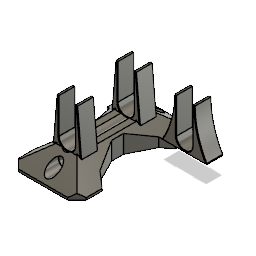
PlayStation TV Display Stand v8 (Autodesk Fusion 360 design; units mm, degrees)
Autodesk Fusion 360 part; units mm, degrees
(part 1 of 2)
sketch "Sketch1" plane through (0, 0, 0) normal (0, 0, 1) x (1, 0, 0)
  line L0 (0, 0) -> (14, 0)
  line L1 (14, 0) -> (14, 35)
  line L2 (14, 35) -> (0, 35)
  line L3 (0, 35) -> (0, 0)
  circle A0 centre (7, 7) radius 7
  line L4 (16, -2) -> (16, 37)
  line L5 (16, 37) -> (-2, 37)
  line L6 (-2, 37) -> (-2, -2)
  line L7 (-2, -2) -> (16, -2)
  line L8 (-2, 35) -> (16, 35)
  dimension "d1" = 14
  dimension "d2" = 35
  dimension "d3" = 2
  constraint horizontal L0
  constraint vertical L1
  constraint horizontal L2
  constraint vertical L3
  constraint coincident L0.start L3.end
  constraint tangent L0 A0
  constraint tangent L1 A0
  constraint tangent L3 A0
  constraint coincident L6 L8.start
  constraint coincident L4 L8.end
  constraint perpendicular L4 L8
  measures "d1" distance of L0.start L0.end
  measures "d2" distance of L0.start L2.end
extrude "Extrude1" add sketch "Sketch1" along normal blind 15 contours L0 L3 A0 | L0 L1 L3 L4 L6 L7 L8 | L0 L1 A0 makes body 1
extrude "Extrude2" add 1 faces at (4, -2, 5) along direction (0, -1, 0) blind 10 on bodies 1 bodies 1
extrude "Extrude3" add 1 faces at (4, -12, 5) along direction (0, -1, 0) blind 5 on bodies 1 bodies 1
sketch "Sketch2" plane through (0, 0, 15) normal (0, 0, 1) x (1, 0, 0)
  line L0 (16, -17) -> (16, 35)
  line L1 (16, 35) -> (14, 35)
  line L2 (14, 35) -> (14, 7)
  arc A0 (0, 7) -> (14, 7) centre (7, 7) ccw
  line L3 (0, 7) -> (0, 35)
  line L4 (0, 35) -> (-2, 35)
  line L5 (-2, 35) -> (-2, -17)
  line L6 (7, 0) -> (7, -4.4)
  circle A1 centre (7, -7) radius 2.6
  line L7 (7, -9.6) -> (7, -14)
  line L8 (16, -17) -> (-2, -17)
  line L9 (-2, -17) -> (-2, -14)
  line L10 (-2, -14) -> (16, -14)
  line L11 (16, -14) -> (16, -17)
  dimension "d10" = 4.4
  dimension "d27" = 5.2
  dimension "d28" = 4.4
  constraint midpoint A0 L6.start
  constraint vertical L6
  constraint coincident L6.end A1
  constraint coincident A1 L7.start
  constraint vertical L7
  constraint horizontal L8
  constraint vertical L9
  constraint horizontal L10
  constraint vertical L11
  constraint coincident L5 L9.end
  constraint coincident L0.start L8.start
  measures "d10" distance of L6.start L6.end
  measures "d27" diameter of A1
  measures "d28" distance of L7.start L7.end
extrude "Extrude4" cut sketch "Sketch2" against normal blind 36 contours L0 L5 L8 L9 L10 L11 bodies 1
sketch "Sketch3" plane through (0, -14, 0) normal (0, -1, 0) x (1, 0, 0)
  line L0 (-2, 0) -> (16, 0)
  line L1 (16, 0) -> (16, 15)
  line L2 (16, 15) -> (-2, 15)
  line L3 (-2, 15) -> (-2, 0)
  line L4 (-2, 7.5) -> (16, 7.5)
  line L5 (7, 7.5) -> (7, 9.3)
  line L6 (7, 9.3) -> (11.6, 9.3)
  line L7 (11.6, 9.3) -> (2.4, 9.3)
  line L8 (2.4, 9.3) -> (2.4, 5.7)
  line L9 (2.4, 5.7) -> (11.6, 5.7)
  line L10 (11.6, 5.7) -> (11.6, 9.3)
  line L11 (-2, 0) -> (16, 0)
  line L12 (16, 0) -> (16, 15)
  line L13 (16, 15) -> (-2, 15)
  line L14 (-2, 15) -> (-2, 0)
  dimension "d15" = 1.8
  dimension "d16" = 4.6
  dimension "d17" = 9.2
  dimension "d18" = 3.6
  constraint midpoint L3 L4.start
  constraint midpoint L1 L4.end
  constraint midpoint L4 L5.start
  constraint perpendicular L4 L5
  constraint perpendicular L5 L6
  constraint horizontal L7
  constraint vertical L8
  constraint horizontal L9
  constraint vertical L10
  measures "d15" distance of L5.start L5.end
  measures "d16" distance of L5.end L6.end
  measures "d17" distance of L6.end L7.end
  measures "d18" distance of L6.end L9.end
extrude "Extrude5" cut sketch "Sketch3" against normal blind 12 contours L4 L5 L7 L8 | L4 L8 L9 L10 | L4 L5 L6 L7 L10 bodies 1
extrude "Extrude9" cut sketch "Sketch2" against normal blind 25 contours A1 bodies 1
extrude "Extrude7" add 1 faces at (-0.6667, 35, 10) along direction (0, 1, 0) blind 2 on bodies 1 bodies 1
extrude "Extrude8" add 1 faces at (15.3333, 35, 10) along direction (0, 1, 0) blind 2 on bodies 1 bodies 1
sketch "Sketch14" plane through (0, 0, 5.7) normal (0, 0, 1) x (1, 0, 0)
  circle A0 centre (7, -7) radius 2.6
  line L0 (2.4, -14) -> (11.6, -14)
  line L1 (11.6, -14) -> (11.6, -2)
  line L2 (11.6, -2) -> (2.4, -2)
  line L3 (2.4, -2) -> (2.4, -14)
  line L4 (2.4, -14) -> (11.6, -14)
  line L5 (11.6, -14) -> (11.6, -2)
  line L6 (11.6, -2) -> (2.4, -2)
  line L7 (2.4, -2) -> (2.4, -14)
  circle A1 centre (7, -7) radius 2.6
  line L8 (3.2, -13.2) -> (10.8, -13.2)
  line L9 (10.8, -13.2) -> (10.8, -2.8)
  line L10 (10.8, -2.8) -> (3.2, -2.8)
  line L11 (3.2, -2.8) -> (3.2, -13.2)
  dimension "d133" = -0.8
  constraint horizontal L4
  constraint vertical L5
  constraint horizontal L6
  constraint vertical L7
  constraint coincident L1.end L2.start
  constraint coincident L0.start L3.end
  constraint concentric A0 A1
extrude "Extrude33" cut sketch "Sketch14" against normal blind 1.2 contours L8 L9 L10 L11 bodies 1
chamfer "Chamfer9" distance 1.2 distance2 3 1 edges at (7, -2.8, 4.5) measured on face at (8.2667, -2.8, 5.3) on bodies 1
chamfer "Chamfer10" distance 1.2 distance2 5 1 edges at (7, -13.2, 4.5) measured on face at (5.7333, -13.2, 5.3) on bodies 1
chamfer "Chamfer11" distance 1.2 distance2 1.49 2 edges at (10.8, -7, 4.5) (3.2, -7, 4.5) measured on face at (10.8, -8.0667, 5.3) measured on face at (3.2, -8.0667, 5.3) on bodies 1
copy_body "CopyPasteBodies1" bodies 1 makes body 2
move_body "Move1" bodies 2 to x (-1, 0, 0) y (0, 1, 0) z (0, 0, -1) at (14, 0, 95.1)
sketch "Sketch4" plane through (0, -14, 0) normal (0, -1, 0) x (1, 0, 0)
  line L0 (11.6, 85.8) -> (2.4, 85.8)
  line L1 (2.4, 85.8) -> (2.4, 89.4)
  line L2 (2.4, 89.4) -> (11.6, 89.4)
  line L3 (11.6, 89.4) -> (11.6, 85.8)
  line L4 (16, 95.1) -> (-2, 95.1)
  line L5 (-2, 95.1) -> (-2, 80.1)
  line L6 (-2, 80.1) -> (16, 80.1)
  line L7 (16, 80.1) -> (16, 95.1)
  line L8 (16, 95.1) -> (-2, 95.1)
  line L9 (-2, 95.1) -> (-2, 30)
  line L10 (-2, 30) -> (16, 30)
  line L11 (16, 30) -> (16, 95.1)
  line L12 (-2, 30) -> (16, 30)
  line L13 (16, 30) -> (16, 45)
  line L14 (16, 45) -> (-2, 45)
  line L15 (-2, 45) -> (-2, 30)
  line L16 (16, 95.1) -> (-2, 95.1)
  line L17 (-2, 95.1) -> (-2, 115.1)
  line L18 (-2, 115.1) -> (16, 115.1)
  line L19 (16, 115.1) -> (16, 95.1)
  line L20 (-2, 30) -> (16, 30)
  line L21 (16, 30) -> (16, 10)
  line L22 (16, 10) -> (-2, 10)
  line L23 (-2, 10) -> (-2, 30)
  line L24 (16, 115.1) -> (36, 115.1)
  line L25 (-2, 10) -> (-22, 10)
  line L26 (-22, 10) -> (-22, 115.1)
  line L27 (-22, 115.1) -> (-2, 115.1)
  line L28 (-2, 115.1) -> (-2, 10)
  line L29 (36, 115.1) -> (16, 115.1)
  line L30 (16, 115.1) -> (16, 10)
  line L31 (16, 10) -> (36, 10)
  line L32 (36, 10) -> (36, 115.1)
  dimension "d31" = 65.1
  dimension "d32" = 15
  dimension "d33" = 20
  dimension "d34" = 18
  dimension "d35" = 20
  dimension "d36" = 20
  dimension "d37" = 20
  constraint horizontal L8
  constraint vertical L9
  constraint horizontal L10
  constraint vertical L11
  constraint coincident L4.start L7.end
  constraint horizontal L12
  constraint vertical L13
  constraint horizontal L14
  constraint vertical L15
  constraint horizontal L16
  constraint vertical L17
  constraint horizontal L18
  constraint vertical L19
  constraint horizontal L20
  constraint vertical L21
  constraint horizontal L22
  constraint vertical L23
  constraint horizontal L24
  constraint horizontal L25
  constraint vertical L26
  constraint horizontal L27
  constraint vertical L28
  constraint horizontal L29
  constraint vertical L30
  constraint horizontal L31
  constraint vertical L32
  measures "d31" distance of L4.start L10.end
  measures "d32" distance of L9.end L14.end
  measures "d33" distance of L4.start L18.end
  measures "d34" distance of L9.end L10.end
  measures "d35" distance of L9.end L22.end
  measures "d36" distance of L18.end L24.end
  measures "d37" distance of L22.end L25.end
move_body "Move3" bodies 1 to x (1, 0, 0) y (0, 1, 0) z (0, 0, 1) at (0, 0, 29.95)
extrude "Extrude10" add sketch "Sketch4" against normal blind 15 separate body contours L7 L11 L13 L19 L21 L24 L29 L30 L31 L32 | L4 L8 L16 L17 L18 L19 L28 L30 | L5 L9 L15 L17 L23 L25 L26 L27 L28 | L6 L9 L11 L14 L28 L30 | L10 L12 L20 L21 L22 L23 L28 L30 makes body 3
extrude "Extrude11" cut sketch "Sketch1" along normal blind 100 and the other way blind -24.95 contours A0 bodies 3
extrude "Extrude12" cut sketch "Sketch2" along normal blind 116 and the other way blind 69 contours A1 bodies 3
sketch "Sketch6" plane through (0, 0, 10) normal (0, 0, -1) x (-1, 0, 0)
  circle A0 centre (-7, -7) radius 2.6
  line L0 (-36, -14) -> (22, -14)
  line L1 (22, -14) -> (22, 1)
  line L2 (22, 1) -> (-36, 1)
  circle A1 centre (-7, -7) radius 4.925
  line L3 (-36, 1) -> (-36, -14)
  dimension "d58" = 9.85
  constraint concentric A0 A1
  measures "d58" diameter of A1
extrude "Extrude14" cut sketch "Sketch6" along normal blind -18 and the other way blind 0 contours A1 bodies 3
sketch "Sketch7" plane through (0, 0, 115.1) normal (0, 0, 1) x (1, 0, 0)
  circle A0 centre (7, -7) radius 2.6
  line L0 (-22, -14) -> (36, -14)
  line L1 (36, 1) -> (-22, 1)
  line L2 (-22, 1) -> (-22, -14)
  circle A1 centre (7, -7) radius 4.925
  line L3 (36, -14) -> (36, 1)
  dimension "d63" = 9.85
  constraint concentric A0 A1
  measures "d63" diameter of A1
extrude "Extrude15" cut sketch "Sketch7" against normal blind 18 contours A1 bodies 3
chamfer "Chamfer1" distance 20 distance2 15 2 edges at (7, 1, 10) (7, 1, 115.1) measured on face at (29.3333, 1, 56.7) measured on face at (29.3333, 1, 56.7) on bodies 3
chamfer "Chamfer2" distance 20 distance2 15 2 edges at (-22, 1, 62.55) (36, 1, 62.55) measured on face at (-15.3333, 1, 68.4) measured on face at (29.3333, 1, 56.7) on bodies 3
move_face "OffsetFaces3" offset -0.25 8 faces at (1.4326, -6.1246, 44.95) (16, 3, 34.95) (1.4326, -6.1246, 29.95) (-2, 3, 34.95) (16, 3, 90.1) (12.5674, -6.1246, 95.1) (12.5674, -6.1246, 80.1) (-2, 3, 90.1) on bodies 1 2
extrude "Extrude16" add 3 faces at (36, -13.999, 80.0653) (29.3333, -14, 56.7) (-22, -13.999, 45.0347) along direction (0, -1, 0) blind 2 on bodies 3 bodies 3
sketch "Sketch5" plane through (0, -16, 0) normal (0, -1, 0) x (1, 0, 0)
  line L0 (-2, 15) -> (16, 15)
  line L1 (16, 15) -> (16, 0)
  line L2 (16, 0) -> (-2, 0)
  line L3 (-2, 0) -> (-2, 15)
  line L4 (-2, 95.1) -> (16, 95.1)
  line L5 (16, 95.1) -> (16, 80.1)
  line L6 (16, 80.1) -> (-2, 80.1)
  line L7 (-2, 80.1) -> (-2, 95.1)
  line L8 (-24.6667, 117.7667) -> (-24.6667, -22.6667)
  line L9 (-24.6667, -22.6667) -> (38.6667, -22.6667)
  line L10 (38.6667, -22.6667) -> (38.6667, 117.7667)
  line L11 (38.6667, 117.7667) -> (-24.6667, 117.7667)
  line L12 (-2, 45) -> (16, 45)
  line L13 (16, 45) -> (16, 30)
  line L14 (16, 30) -> (-2, 30)
  line L15 (-2, 30) -> (-2, 45)
  line L16 (-2, 95.1) -> (16, 95.1)
  line L17 (16, 95.1) -> (16, 80.1)
  line L18 (16, 80.1) -> (-2, 80.1)
  line L19 (-2, 80.1) -> (-2, 95.1)
  line L20 (-22, 115.1) -> (-22, 10)
  line L21 (-22, 10) -> (36, 10)
  line L22 (36, 115.1) -> (-22, 115.1)
  line L23 (36, 10) -> (36, 115.1)
extrude "Extrude13" add sketch "Sketch5" against normal blind 1.75 contours L4 L5 L6 L7 L16 L17 L18 L19 | L12 L13 L14 L15 bodies 3
chamfer "Chamfer3" distance 2 angle 45 1 edges at (4.5759, -7.9402, 97.1) on bodies 3
chamfer "Chamfer4" distance 2 angle 45 1 edges at (4.5759, -6.0598, 28) on bodies 3
sketch "Sketch8" plane through (0, 0, 45) normal (0, 0, -1) x (-1, 0, 0)
  line L0 (2, -14.25) -> (2, 1)
  line L1 (2, 1) -> (-3.3944, 1)
  arc A0 (-10.6056, 1) -> (-3.3944, 1) centre (-7, 7) ccw
  line L2 (-16, 1) -> (-16, -14.25)
  circle A1 centre (-7, -7) radius 2.6
  line L3 (-16, -14.25) -> (2, -14.25)
  line L4 (-10.6056, 1) -> (-16, 1)
extrude "Extrude17" add sketch "Sketch8" against normal blind 35.1 contours A1 bodies 3
sketch "Sketch9" plane through (0, 0, 30.2) normal (0, 0, -1) x (-1, 0, 0)
  circle A0 centre (-7, -7) radius 2.6
  line L0 (-15.75, -14) -> (1.75, -14)
  line L1 (1.75, -14) -> (1.75, 37)
  line L2 (1.75, 37) -> (0, 37)
  line L3 (0, 37) -> (0, 7)
  arc A1 (-14, 7) -> (0, 7) centre (-7, 7) ccw
  line L4 (-14, 7) -> (-14, 37)
  line L5 (-14, 37) -> (-15.75, 37)
  line L6 (-15.75, 37) -> (-15.75, -14)
  line L7 (-15.75, -14) -> (-36, -14)
  line L8 (-15.75, 37) -> (-19.0909, -1.1867)
  line L9 (-15.75, 37) -> (22.8917, 37) construction
  line L10 (1.75, -14) -> (22, -14)
  line L11 (1.75, -14) -> (1.75, 1)
  line L12 (1.75, 37) -> (5.1179, -1.4947)
  line L13 (1.75, 37) -> (40.3917, 37) construction
  line L14 (1.75, 1) -> (2, 1)
  line L15 (2, 1) -> (22, -14)
  line L16 (-15.75, -14) -> (-15.75, 1)
  line L17 (-15.75, 1) -> (-16, 1)
  line L18 (-16, 1) -> (-36, -14)
  line L19 (-19.0909, -1.1867) -> (-19.1919, -2.3414)
  dimension "d72" = 20.25
  dimension "d73" = 95
  dimension "d76" = 20.25
  dimension "d77" = 15
  dimension "d78" = 85
  dimension "d84" = 0.25
  dimension "d85" = 15
  dimension "d86" = 0.25
  constraint coincident L0.start L6.end
  constraint perpendicular L6 L7
  constraint horizontal L9
  constraint coincident L5.end L6.start
  constraint coincident L0.end L1.start
  constraint perpendicular L1 L10
  constraint perpendicular L10 L11
  constraint horizontal L13
  constraint coincident L1.end L2.start
  constraint perpendicular L1 L14
  constraint perpendicular L7 L16
  constraint perpendicular L16 L17
  constraint parallel L8 L19
  measures "d72" distance of L0.start L7.end
  measures "d73" angle of L8 L9
  measures "d76" distance of L0.end L10.end
  measures "d77" distance of L0.end L11.end
  measures "d78" angle of L12 L13
  measures "d84" distance of L11.end L14.end
  measures "d85" distance of L0.start L16.end
  measures "d86" distance of L16.end L17.end
extrude "Extrude19" add sketch "Sketch9" along normal blind -50.15 and the other way blind 64.65 contours L6 L8 L17 L18 L19 | L1 L12 L14 L15 bodies 2
extrude "Extrude18" add sketch "Sketch9" against normal blind 14.5 contours L6 L8 L17 L18 L19 | L1 L12 L14 L15 bodies 1
move_face "OffsetFaces6" offset -0.25 4 faces at (-3.0344, 0.2242, 39.8667) (17.0344, 0.2242, 39.8667) (17.0344, 0.2242, 85.1833) (-3.0344, 0.2242, 90.0167) on bodies 1 2
move_face "OffsetFaces7" offset -0.25 4 faces at (-1.9722, 1, 39.8667) (15.9722, 1, 39.8667) (15.9722, 1, 85.1833) (-2.1944, 1, 85.1833) on bodies 1 2
sketch "Sketch10" plane through (36, 0, 0) normal (1, 0, 0) x (0, 0, -1)
  line L0 (-115.1, -16) -> (20, -16)
  line L1 (-115.1, -16) -> (-10, -16)
  line L2 (-10, -16) -> (-10, -14)
  line L3 (-115.1, -14) -> (-115.1, -16)
  line L4 (-115.1, -14) -> (-87.6, -14)
  line L5 (-87.6, -14) -> (-87.6, -3)
  line L6 (-87.6, -3) -> (-115.1, -3)
  line L7 (-115.1, -3) -> (-115.1, -14)
  line L8 (-10, -14) -> (-37.5, -14)
  line L9 (-37.5, -14) -> (-37.5, -3)
  line L10 (-37.5, -3) -> (-10, -3)
  line L11 (-10, -3) -> (-10, -14)
  line L12 (-37.5, -14) -> (-37.5, 6)
  line L13 (-37.5, 6) -> (-87.6, 6)
  line L14 (-87.6, 6) -> (-87.6, -14)
  line L15 (-87.6, 6) -> (-37.5, 6)
  line L16 (-37.5, 6) -> (-37.5, -16)
  line L17 (-37.5, -16) -> (-87.6, -16)
  line L18 (-87.6, -16) -> (-87.6, 6)
  dimension "d148" = 105.1
  dimension "d149" = 27.5
  dimension "d150" = 11
  dimension "d151" = 27.5
  dimension "d152" = 11
  dimension "d153" = 20
  dimension "d154" = 22
  constraint horizontal L1
  constraint vertical L2
  constraint vertical L3
  constraint horizontal L4
  constraint vertical L5
  constraint horizontal L6
  constraint vertical L7
  constraint horizontal L8
  constraint vertical L9
  constraint horizontal L10
  constraint vertical L11
  constraint vertical L12
  constraint horizontal L13
  constraint vertical L14
  constraint horizontal L15
  constraint vertical L16
  constraint horizontal L17
  constraint vertical L18
  measures "d148" distance of L0.start L1.end
  measures "d149" distance of L3.start L4.end
  measures "d150" distance of L3.start L6.end
  measures "d151" distance of L2.end L8.end
  measures "d152" distance of L2.end L10.end
  measures "d153" distance of L4.end L13.end
  measures "d154" distance of L13.end L17.end
extrude "Extrude20" cut sketch "Sketch10" against normal blind 18 contours L0 L1 L5 L9 L12 L13 L14 L15 L16 L17 L18 bodies 3
extrude "Extrude21" cut 1 faces at (18, -5.6647, 70.9) along direction (1, 0, 0) blind -75 and the other way blind 22 on bodies 3 bodies 3
chamfer "Chamfer5" distance 20 distance2 10 2 edges at (-4, -8.25, 87.6) (-4, -8.25, 37.5) measured on face at (-4, -5.6647, 70.9) measured on face at (-4, -5.6647, 70.9) on bodies 3
chamfer "Chamfer12" distance 6 distance2 8 2 edges at (-22, -15, 37.5) (-22, -15, 87.6) measured on face at (-22, -15.3323, 19.168) measured on face at (-22, -15.3323, 105.932) on bodies 3
chamfer "Chamfer6" distance 10 distance2 20 2 edges at (18, -8.25, 37.5) (18, -8.25, 87.6) measured on face at (24, -10.1647, 37.5) measured on face at (24, -10.1647, 87.6) on bodies 3
chamfer "Chamfer13" distance 6 distance2 8 2 edges at (36, -15, 87.6) (36, -15, 37.5) measured on face at (36, -15.3323, 105.932) measured on face at (36, -15.3323, 19.168) on bodies 3
chamfer "Chamfer14" distance 8 distance2 8 4 edges at (36, -15, 115.1) (-22, -15, 115.1) (-22, -15, 10) (36, -15, 10) measured on face at (36, -15.3323, 107.9316) measured on face at (-2.6667, -14.6667, 115.1) measured on face at (-22, -15.3323, 17.1684) measured on face at (-2.6667, -14.6667, 10) on bodies 3
copy_body "CopyPasteBodies2" bodies 1 makes body 4
move_body "Move2" bodies 4 to x (1, 0, 0) y (0, 1, 0) z (0, 0, 1) at (50, 0, 0)
sketch "Sketch11" plane through (0, 0, 44.7) normal (0, 0, 1) x (1, 0, 0)
  circle A0 centre (57, -7) radius 2.6
  line L0 (48.25, -14) -> (65.75, -14)
  line L1 (65.75, -14) -> (65.75, 1.25)
  line L2 (65.75, 1.25) -> (66.0833, 1.25)
  line L3 (66.0833, 1.25) -> (69.074, -0.993)
  line L4 (69.074, -0.993) -> (65.75, 37)
  line L5 (65.75, 37) -> (64, 37)
  line L6 (64, 37) -> (64, 7)
  arc A1 (50, 7) -> (64, 7) centre (57, 7) ccw
  line L7 (50, 7) -> (50, 37)
  line L8 (50, 37) -> (48.25, 37)
  line L9 (48.25, 37) -> (44.926, -0.993)
  line L10 (44.926, -0.993) -> (47.9167, 1.25)
  line L11 (47.9167, 1.25) -> (48.25, 1.25)
  line L12 (48.25, 1.25) -> (48.25, -14)
  line L13 (44.926, -0.993) -> (69.074, -0.993)
  constraint coincident L9.end L10.start
  constraint coincident L3.end L4.start
extrude "Extrude22" add sketch "Sketch11" against normal blind 14.5 contours L10 L11 L12 L13 | L1 L2 L3 L13 bodies 4
extrude "Extrude23" cut sketch "Sketch11" against normal blind 42 contours L0 L1 L12 L13 bodies 4
extrude "Extrude24" cut 1 faces at (52.9753, -0.993, 35.0333) along direction (0, 1, 0) blind 0.593 on bodies 4 bodies 4
sketch "Sketch12" plane through (0, 0, 44.7) normal (0, 0, 1) x (1, 0, 0)
  line L0 (44.9779, -0.4) -> (69.0221, -0.4)
  line L1 (69.0221, -0.4) -> (65.75, 37)
  line L2 (65.75, 37) -> (64, 37)
  line L3 (64, 37) -> (64, 7)
  arc A0 (50, 7) -> (64, 7) centre (57, 7) ccw
  line L4 (50, 7) -> (50, 37)
  line L5 (50, 37) -> (48.25, 37)
  line L6 (48.25, 37) -> (44.9779, -0.4)
  line L7 (48.25, 37) -> (48.25, 36)
  line L8 (48.25, 36) -> (48.25, -0.4)
  line L9 (48.25, -0.4) -> (38.25, -0.4)
  line L10 (65.75, 37) -> (65.75, -0.4)
  line L11 (65.75, -0.4) -> (75.75, -0.4)
  arc A1 (38.25, -0.4) -> (48.25, 37) centre (-26.6879, 37) ccw
  arc A2 (65.75, 37) -> (75.75, -0.4) centre (140.6879, 37) ccw
  dimension "d111" = 10
  dimension "d112" = 10
  constraint coincident L5.end L6.start
  constraint perpendicular L5 L7
  constraint coincident L0 L8.end
  constraint perpendicular L0 L8
  constraint perpendicular L8 L9
  constraint coincident L1.end L2.start
  constraint coincident L0 L10.end
  constraint perpendicular L0 L10
  constraint perpendicular L10 L11
  constraint tangent L8 A1
  constraint tangent L10 A2
  measures "d111" distance of L8.end L9.end
  measures "d112" distance of L10.end L11.end
extrude "Extrude26" add sketch "Sketch12" against normal blind 14.5 contours L6 L9 A1 | L1 L11 A2 bodies 4
extrude "Extrude27" cut sketch "Sketch12" against normal blind 14.5 contours L6 A1 | L1 A2 bodies 4
extrude "Extrude28" add 1 faces at (50.75, -0.4, 39.8667) along direction (0, -1, 0) blind 1 on bodies 4 bodies 4
sketch "Sketch16" plane through (0, -16, 0) normal (0, -1, 0) x (1, 0, 0)
  line L0 (28, 10) -> (36, 18)
  line L1 (36, 18) -> (36, 31.5)
  line L2 (36, 31.5) -> (28, 37.5)
  line L3 (28, 37.5) -> (18, 57.5)
  line L4 (18, 57.5) -> (18, 67.6)
  line L5 (18, 67.6) -> (28, 87.6)
  line L6 (28, 87.6) -> (36, 93.6)
  line L7 (36, 93.6) -> (36, 107.1)
  line L8 (36, 107.1) -> (28, 115.1)
  line L9 (28, 115.1) -> (-14, 115.1)
  line L10 (-14, 115.1) -> (-22, 107.1)
  line L11 (-22, 107.1) -> (-22, 93.6)
  line L12 (-22, 93.6) -> (-14, 87.6)
  line L13 (-14, 87.6) -> (-4, 67.6)
  line L14 (-4, 67.6) -> (-4, 57.5)
  line L15 (-4, 57.5) -> (-14, 37.5)
  line L16 (-14, 37.5) -> (-22, 31.5)
  line L17 (-22, 31.5) -> (-22, 18)
  line L18 (-22, 18) -> (-14, 10)
  line L19 (-14, 10) -> (28, 10)
  line L20 (1.0417, 0) -> (1.0417, -0.2083)
  line L21 (1.0417, -0.2083) -> (0.8333, -0.2083)
  line L22 (0.8333, -0.2083) -> (0.8333, -0.4167)
  line L23 (0.8333, -0.4167) -> (0.625, -0.4167)
  line L24 (0.625, -0.4167) -> (0.625, -0.625)
  line L25 (0.625, -0.625) -> (0.4167, -0.625)
  line L26 (0.4167, -0.625) -> (0.4167, -0.8333)
  line L27 (0.4167, -0.8333) -> (0.2083, -0.8333)
  line L28 (0.2083, -0.8333) -> (0.2083, -1.0417)
  line L29 (0.2083, -1.0417) -> (0, -1.0417)
  line L30 (0, -1.0417) -> (0, -1.4583)
  line L31 (0, -1.4583) -> (1.25, -1.4583)
  line L32 (1.25, -1.4583) -> (1.25, -4.5833)
  line L33 (1.25, -4.5833) -> (0, -4.5833)
  line L34 (0, -4.5833) -> (0, -5.625)
  line L35 (0, -5.625) -> (3.125, -5.625)
  line L36 (3.125, -5.625) -> (3.125, -4.5833)
  line L37 (3.125, -4.5833) -> (2.2917, -4.5833)
  line L38 (2.2917, -4.5833) -> (2.2917, 0)
  line L39 (2.2917, 0) -> (1.0417, 0)
  line L40 (4.375, 0) -> (4.375, -0.2083)
  line L41 (4.375, -0.2083) -> (4.1667, -0.2083)
  line L42 (4.1667, -0.2083) -> (4.1667, -0.4167)
  line L43 (4.1667, -0.4167) -> (3.9583, -0.4167)
  line L44 (3.9583, -0.4167) -> (3.9583, -0.625)
  line L45 (3.9583, -0.625) -> (3.75, -0.625)
  line L46 (3.75, -0.625) -> (3.75, -0.8333)
  line L47 (3.75, -0.8333) -> (3.5417, -0.8333)
  line L48 (3.5417, -0.8333) -> (3.5417, -4.7917)
  line L49 (3.5417, -4.7917) -> (3.75, -4.7917)
  line L50 (3.75, -4.7917) -> (3.75, -5)
  line L51 (3.75, -5) -> (3.9583, -5)
  line L52 (3.9583, -5) -> (3.9583, -5.2083)
  line L53 (3.9583, -5.2083) -> (4.1667, -5.2083)
  line L54 (4.1667, -5.2083) -> (4.1667, -5.4167)
  line L55 (4.1667, -5.4167) -> (4.375, -5.4167)
  line L56 (4.375, -5.4167) -> (4.375, -5.625)
  line L57 (4.375, -5.625) -> (6.25, -5.625)
  line L58 (6.25, -5.625) -> (6.25, -5.4167)
  line L59 (6.25, -5.4167) -> (6.4583, -5.4167)
  line L60 (6.4583, -5.4167) -> (6.4583, -5.2083)
  line L61 (6.4583, -5.2083) -> (6.6667, -5.2083)
  line L62 (6.6667, -5.2083) -> (6.6667, -5)
  line L63 (6.6667, -5) -> (6.875, -5)
  line L64 (6.875, -5) -> (6.875, -3.125)
  line L65 (6.875, -3.125) -> (6.6667, -3.125)
  line L66 (6.6667, -3.125) -> (6.6667, -2.9167)
  line L67 (6.6667, -2.9167) -> (6.4583, -2.9167)
  line L68 (6.4583, -2.9167) -> (6.4583, -2.7083)
  line L69 (6.4583, -2.7083) -> (6.25, -2.7083)
  line L70 (6.25, -2.7083) -> (6.25, -2.5)
  line L71 (6.25, -2.5) -> (6.0417, -2.5)
  line L72 (6.0417, -2.5) -> (6.0417, -2.2917)
  line L73 (6.0417, -2.2917) -> (4.7917, -2.2917)
  line L74 (4.7917, -2.2917) -> (4.7917, -2.5)
  line L75 (4.7917, -2.5) -> (4.5833, -2.5)
  line L76 (4.5833, -2.5) -> (4.5833, -1.6667)
  line L77 (4.5833, -1.6667) -> (4.7917, -1.6667)
  line L78 (4.7917, -1.6667) -> (4.7917, -1.4583)
  line L79 (4.7917, -1.4583) -> (5, -1.4583)
  line L80 (5, -1.4583) -> (5, -1.25)
  line L81 (5, -1.25) -> (5.625, -1.25)
  line L82 (5.625, -1.25) -> (5.625, -1.4583)
  line L83 (5.625, -1.4583) -> (5.8333, -1.4583)
  line L84 (5.8333, -1.4583) -> (5.8333, -1.875)
  line L85 (5.8333, -1.875) -> (6.875, -1.875)
  line L86 (6.875, -1.875) -> (6.875, -0.8333)
  line L87 (6.875, -0.8333) -> (6.6667, -0.8333)
  line L88 (6.6667, -0.8333) -> (6.6667, -0.625)
  line L89 (6.6667, -0.625) -> (6.4583, -0.625)
  line L90 (6.4583, -0.625) -> (6.4583, -0.4167)
  line L91 (6.4583, -0.4167) -> (6.25, -0.4167)
  line L92 (6.25, -0.4167) -> (6.25, -0.2083)
  line L93 (6.25, -0.2083) -> (6.0417, -0.2083)
  line L94 (6.0417, -0.2083) -> (6.0417, 0)
  line L95 (6.0417, 0) -> (4.375, 0)
  line L96 (8.125, 0) -> (8.125, -5.625)
  line L97 (8.125, -5.625) -> (10, -5.625)
  line L98 (10, -5.625) -> (10, -5.4167)
  line L99 (10, -5.4167) -> (10.2083, -5.4167)
  line L100 (10.2083, -5.4167) -> (10.2083, -5.2083)
  line L101 (10.2083, -5.2083) -> (10.4167, -5.2083)
  line L102 (10.4167, -5.2083) -> (10.4167, -5)
  line L103 (10.4167, -5) -> (10.625, -5)
  line L104 (10.625, -5) -> (10.625, -3.125)
  line L105 (10.625, -3.125) -> (10.4167, -3.125)
  line L106 (10.4167, -3.125) -> (10.4167, -2.9167)
  line L107 (10.4167, -2.9167) -> (10.2083, -2.9167)
  line L108 (10.2083, -2.9167) -> (10.2083, -2.7083)
  line L109 (10.2083, -2.7083) -> (10.4167, -2.7083)
  line L110 (10.4167, -2.7083) -> (10.4167, -2.5)
  line L111 (10.4167, -2.5) -> (10.625, -2.5)
  line L112 (10.625, -2.5) -> (10.625, -0.625)
  line L113 (10.625, -0.625) -> (10.4167, -0.625)
  line L114 (10.4167, -0.625) -> (10.4167, -0.4167)
  line L115 (10.4167, -0.4167) -> (10.2083, -0.4167)
  line L116 (10.2083, -0.4167) -> (10.2083, -0.2083)
  line L117 (10.2083, -0.2083) -> (10, -0.2083)
  line L118 (10, -0.2083) -> (10, 0)
  line L119 (10, 0) -> (8.125, 0)
  line L120 (11.0417, 0) -> (11.0417, -1.0417)
  line L121 (11.0417, -1.0417) -> (11.875, -1.0417)
  line L122 (11.875, -1.0417) -> (11.875, -4.5833)
  line L123 (11.875, -4.5833) -> (11.0417, -4.5833)
  line L124 (11.0417, -4.5833) -> (11.0417, -5.625)
  line L125 (11.0417, -5.625) -> (13.9583, -5.625)
  line L126 (13.9583, -5.625) -> (13.9583, -4.5833)
  line L127 (13.9583, -4.5833) -> (13.125, -4.5833)
  line L128 (13.125, -4.5833) -> (13.125, -1.0417)
  line L129 (13.125, -1.0417) -> (13.9583, -1.0417)
  line L130 (13.9583, -1.0417) -> (13.9583, 0)
  line L131 (13.9583, 0) -> (11.0417, 0)
  line L132 (14.375, 0) -> (14.375, -1.0417)
  line L133 (14.375, -1.0417) -> (15.2083, -1.0417)
  line L134 (15.2083, -1.0417) -> (15.2083, -5.625)
  line L135 (15.2083, -5.625) -> (16.4583, -5.625)
  line L136 (16.4583, -5.625) -> (16.4583, -1.0417)
  line L137 (16.4583, -1.0417) -> (17.2917, -1.0417)
  line L138 (17.2917, -1.0417) -> (17.2917, 0)
  line L139 (17.2917, 0) -> (14.375, 0)
  line L140 (2.0833, -0.2083) -> (2.0833, -4.7917)
  line L141 (2.0833, -4.7917) -> (2.9167, -4.7917)
  line L142 (2.9167, -4.7917) -> (2.9167, -5.4167)
  line L143 (2.9167, -5.4167) -> (0.2083, -5.4167)
  line L144 (0.2083, -5.4167) -> (0.2083, -4.7917)
  line L145 (0.2083, -4.7917) -> (1.4583, -4.7917)
  line L146 (1.4583, -4.7917) -> (1.4583, -1.25)
  line L147 (1.4583, -1.25) -> (0.4167, -1.25)
  line L148 (0.4167, -1.25) -> (0.4167, -1.0417)
  line L149 (0.4167, -1.0417) -> (0.625, -1.0417)
  line L150 (0.625, -1.0417) -> (0.625, -0.8333)
  line L151 (0.625, -0.8333) -> (0.8333, -0.8333)
  line L152 (0.8333, -0.8333) -> (0.8333, -0.625)
  line L153 (0.8333, -0.625) -> (1.0417, -0.625)
  line L154 (1.0417, -0.625) -> (1.0417, -0.4167)
  line L155 (1.0417, -0.4167) -> (1.25, -0.4167)
  line L156 (1.25, -0.4167) -> (1.25, -0.2083)
  line L157 (1.25, -0.2083) -> (2.0833, -0.2083)
  line L158 (5.8333, -0.2083) -> (5.8333, -0.4167)
  line L159 (5.8333, -0.4167) -> (6.0417, -0.4167)
  line L160 (6.0417, -0.4167) -> (6.0417, -0.625)
  line L161 (6.0417, -0.625) -> (6.25, -0.625)
  line L162 (6.25, -0.625) -> (6.25, -0.8333)
  line L163 (6.25, -0.8333) -> (6.4583, -0.8333)
  line L164 (6.4583, -0.8333) -> (6.4583, -1.0417)
  line L165 (6.4583, -1.0417) -> (6.6667, -1.0417)
  line L166 (6.6667, -1.0417) -> (6.6667, -1.6667)
  line L167 (6.6667, -1.6667) -> (6.0417, -1.6667)
  line L168 (6.0417, -1.6667) -> (6.0417, -1.25)
  line L169 (6.0417, -1.25) -> (5.8333, -1.25)
  line L170 (5.8333, -1.25) -> (5.8333, -1.0417)
  line L171 (5.8333, -1.0417) -> (4.7917, -1.0417)
  line L172 (4.7917, -1.0417) -> (4.7917, -1.25)
  line L173 (4.7917, -1.25) -> (4.5833, -1.25)
  line L174 (4.5833, -1.25) -> (4.5833, -1.4583)
  line L175 (4.5833, -1.4583) -> (4.375, -1.4583)
  line L176 (4.375, -1.4583) -> (4.375, -2.9167)
  line L177 (4.375, -2.9167) -> (4.7917, -2.9167)
  line L178 (4.7917, -2.9167) -> (4.7917, -2.7083)
  line L179 (4.7917, -2.7083) -> (5, -2.7083)
  line L180 (5, -2.7083) -> (5, -2.5)
  line L181 (5, -2.5) -> (5.8333, -2.5)
  line L182 (5.8333, -2.5) -> (5.8333, -2.7083)
  line L183 (5.8333, -2.7083) -> (6.0417, -2.7083)
  line L184 (6.0417, -2.7083) -> (6.0417, -2.9167)
  line L185 (6.0417, -2.9167) -> (6.25, -2.9167)
  line L186 (6.25, -2.9167) -> (6.25, -3.125)
  line L187 (6.25, -3.125) -> (6.4583, -3.125)
  line L188 (6.4583, -3.125) -> (6.4583, -3.3333)
  line L189 (6.4583, -3.3333) -> (6.6667, -3.3333)
  line L190 (6.6667, -3.3333) -> (6.6667, -4.7917)
  line L191 (6.6667, -4.7917) -> (6.4583, -4.7917)
  line L192 (6.4583, -4.7917) -> (6.4583, -5)
  line L193 (6.4583, -5) -> (6.25, -5)
  line L194 (6.25, -5) -> (6.25, -5.2083)
  line L195 (6.25, -5.2083) -> (6.0417, -5.2083)
  line L196 (6.0417, -5.2083) -> (6.0417, -5.4167)
  line L197 (6.0417, -5.4167) -> (4.5833, -5.4167)
  line L198 (4.5833, -5.4167) -> (4.5833, -5.2083)
  line L199 (4.5833, -5.2083) -> (4.375, -5.2083)
  line L200 (4.375, -5.2083) -> (4.375, -5)
  line L201 (4.375, -5) -> (4.1667, -5)
  line L202 (4.1667, -5) -> (4.1667, -4.7917)
  line L203 (4.1667, -4.7917) -> (3.9583, -4.7917)
  line L204 (3.9583, -4.7917) -> (3.9583, -4.5833)
  line L205 (3.9583, -4.5833) -> (3.75, -4.5833)
  line L206 (3.75, -4.5833) -> (3.75, -1.0417)
  line L207 (3.75, -1.0417) -> (3.9583, -1.0417)
  line L208 (3.9583, -1.0417) -> (3.9583, -0.8333)
  line L209 (3.9583, -0.8333) -> (4.1667, -0.8333)
  line L210 (4.1667, -0.8333) -> (4.1667, -0.625)
  line L211 (4.1667, -0.625) -> (4.375, -0.625)
  line L212 (4.375, -0.625) -> (4.375, -0.4167)
  line L213 (4.375, -0.4167) -> (4.5833, -0.4167)
  line L214 (4.5833, -0.4167) -> (4.5833, -0.2083)
  line L215 (4.5833, -0.2083) -> (5.8333, -0.2083)
  line L216 (9.7917, -0.2083) -> (9.7917, -0.4167)
  line L217 (9.7917, -0.4167) -> (10, -0.4167)
  line L218 (10, -0.4167) -> (10, -0.625)
  line L219 (10, -0.625) -> (10.2083, -0.625)
  line L220 (10.2083, -0.625) -> (10.2083, -0.8333)
  line L221 (10.2083, -0.8333) -> (10.4167, -0.8333)
  line L222 (10.4167, -0.8333) -> (10.4167, -2.2917)
  line L223 (10.4167, -2.2917) -> (10.2083, -2.2917)
  line L224 (10.2083, -2.2917) -> (10.2083, -2.5)
  line L225 (10.2083, -2.5) -> (9.5833, -2.5)
  line L226 (9.5833, -2.5) -> (9.5833, -2.7083)
  line L227 (9.5833, -2.7083) -> (9.7917, -2.7083)
  line L228 (9.7917, -2.7083) -> (9.7917, -2.9167)
  line L229 (9.7917, -2.9167) -> (10, -2.9167)
  line L230 (10, -2.9167) -> (10, -3.125)
  line L231 (10, -3.125) -> (10.2083, -3.125)
  line L232 (10.2083, -3.125) -> (10.2083, -3.3333)
  line L233 (10.2083, -3.3333) -> (10.4167, -3.3333)
  line L234 (10.4167, -3.3333) -> (10.4167, -4.7917)
  line L235 (10.4167, -4.7917) -> (10.2083, -4.7917)
  line L236 (10.2083, -4.7917) -> (10.2083, -5)
  line L237 (10.2083, -5) -> (10, -5)
  line L238 (10, -5) -> (10, -5.2083)
  line L239 (10, -5.2083) -> (9.7917, -5.2083)
  line L240 (9.7917, -5.2083) -> (9.7917, -5.4167)
  line L241 (9.7917, -5.4167) -> (8.3333, -5.4167)
  line L242 (8.3333, -5.4167) -> (8.3333, -0.2083)
  line L243 (8.3333, -0.2083) -> (9.7917, -0.2083)
  line L244 (13.75, -0.2083) -> (13.75, -0.8333)
  line L245 (13.75, -0.8333) -> (12.9167, -0.8333)
  line L246 (12.9167, -0.8333) -> (12.9167, -4.7917)
  line L247 (12.9167, -4.7917) -> (13.75, -4.7917)
  line L248 (13.75, -4.7917) -> (13.75, -5.4167)
  line L249 (13.75, -5.4167) -> (11.25, -5.4167)
  line L250 (11.25, -5.4167) -> (11.25, -4.7917)
  line L251 (11.25, -4.7917) -> (12.0833, -4.7917)
  line L252 (12.0833, -4.7917) -> (12.0833, -0.8333)
  line L253 (12.0833, -0.8333) -> (11.25, -0.8333)
  line L254 (11.25, -0.8333) -> (11.25, -0.2083)
  line L255 (11.25, -0.2083) -> (13.75, -0.2083)
  line L256 (17.0833, -0.2083) -> (17.0833, -0.8333)
  line L257 (17.0833, -0.8333) -> (16.25, -0.8333)
  line L258 (16.25, -0.8333) -> (16.25, -5.4167)
  line L259 (16.25, -5.4167) -> (15.4167, -5.4167)
  line L260 (15.4167, -5.4167) -> (15.4167, -0.8333)
  line L261 (15.4167, -0.8333) -> (14.5833, -0.8333)
  line L262 (14.5833, -0.8333) -> (14.5833, -0.2083)
  line L263 (14.5833, -0.2083) -> (17.0833, -0.2083)
  line L264 (8.75, -0.625) -> (8.75, -2.0833)
  line L265 (8.75, -2.0833) -> (9.5833, -2.0833)
  line L266 (9.5833, -2.0833) -> (9.5833, -1.875)
  line L267 (9.5833, -1.875) -> (9.7917, -1.875)
  line L268 (9.7917, -1.875) -> (9.7917, -0.8333)
  line L269 (9.7917, -0.8333) -> (9.5833, -0.8333)
  line L270 (9.5833, -0.8333) -> (9.5833, -0.625)
  line L271 (9.5833, -0.625) -> (8.75, -0.625)
  line L272 (9.375, -0.8333) -> (9.375, -1.0417)
  line L273 (9.375, -1.0417) -> (9.5833, -1.0417)
  line L274 (9.5833, -1.0417) -> (9.5833, -1.6667)
  line L275 (9.5833, -1.6667) -> (9.375, -1.6667)
  line L276 (9.375, -1.6667) -> (9.375, -1.875)
  line L277 (9.375, -1.875) -> (8.9583, -1.875)
  line L278 (8.9583, -1.875) -> (8.9583, -0.8333)
  line L279 (8.9583, -0.8333) -> (9.375, -0.8333)
  line L280 (4.7917, -3.125) -> (4.7917, -3.3333)
  line L281 (4.7917, -3.3333) -> (4.5833, -3.3333)
  line L282 (4.5833, -3.3333) -> (4.5833, -3.5417)
  line L283 (4.5833, -3.5417) -> (4.375, -3.5417)
  line L284 (4.375, -3.5417) -> (4.375, -4.5833)
  line L285 (4.375, -4.5833) -> (4.5833, -4.5833)
  line L286 (4.5833, -4.5833) -> (4.5833, -4.7917)
  line L287 (4.5833, -4.7917) -> (4.7917, -4.7917)
  line L288 (4.7917, -4.7917) -> (4.7917, -5)
  line L289 (4.7917, -5) -> (5.625, -5)
  line L290 (5.625, -5) -> (5.625, -4.7917)
  line L291 (5.625, -4.7917) -> (5.8333, -4.7917)
  line L292 (5.8333, -4.7917) -> (5.8333, -4.5833)
  line L293 (5.8333, -4.5833) -> (6.0417, -4.5833)
  line L294 (6.0417, -4.5833) -> (6.0417, -3.5417)
  line L295 (6.0417, -3.5417) -> (5.8333, -3.5417)
  line L296 (5.8333, -3.5417) -> (5.8333, -3.3333)
  line L297 (5.8333, -3.3333) -> (5.625, -3.3333)
  line L298 (5.625, -3.3333) -> (5.625, -3.125)
  line L299 (5.625, -3.125) -> (4.7917, -3.125)
  line L300 (8.75, -3.125) -> (8.75, -4.7917)
  line L301 (8.75, -4.7917) -> (9.5833, -4.7917)
  line L302 (9.5833, -4.7917) -> (9.5833, -4.5833)
  line L303 (9.5833, -4.5833) -> (9.7917, -4.5833)
  line L304 (9.7917, -4.5833) -> (9.7917, -3.3333)
  line L305 (9.7917, -3.3333) -> (9.5833, -3.3333)
  line L306 (9.5833, -3.3333) -> (9.5833, -3.125)
  line L307 (9.5833, -3.125) -> (8.75, -3.125)
  line L308 (5.4167, -3.3333) -> (5.4167, -3.5417)
  line L309 (5.4167, -3.5417) -> (5.625, -3.5417)
  line L310 (5.625, -3.5417) -> (5.625, -3.75)
  line L311 (5.625, -3.75) -> (5.8333, -3.75)
  line L312 (5.8333, -3.75) -> (5.8333, -4.375)
  line L313 (5.8333, -4.375) -> (5.625, -4.375)
  line L314 (5.625, -4.375) -> (5.625, -4.5833)
  line L315 (5.625, -4.5833) -> (5.4167, -4.5833)
  line L316 (5.4167, -4.5833) -> (5.4167, -4.7917)
  line L317 (5.4167, -4.7917) -> (5, -4.7917)
  line L318 (5, -4.7917) -> (5, -4.5833)
  line L319 (5, -4.5833) -> (4.7917, -4.5833)
  line L320 (4.7917, -4.5833) -> (4.7917, -4.375)
  line L321 (4.7917, -4.375) -> (4.5833, -4.375)
  line L322 (4.5833, -4.375) -> (4.5833, -3.75)
  line L323 (4.5833, -3.75) -> (4.7917, -3.75)
  line L324 (4.7917, -3.75) -> (4.7917, -3.5417)
  line L325 (4.7917, -3.5417) -> (5, -3.5417)
  line L326 (5, -3.5417) -> (5, -3.3333)
  line L327 (5, -3.3333) -> (5.4167, -3.3333)
  line L328 (9.375, -3.3333) -> (9.375, -3.5417)
  line L329 (9.375, -3.5417) -> (9.5833, -3.5417)
  line L330 (9.5833, -3.5417) -> (9.5833, -4.375)
  line L331 (9.5833, -4.375) -> (9.375, -4.375)
  line L332 (9.375, -4.375) -> (9.375, -4.5833)
  line L333 (9.375, -4.5833) -> (8.9583, -4.5833)
  line L334 (8.9583, -4.5833) -> (8.9583, -3.3333)
  line L335 (8.9583, -3.3333) -> (9.375, -3.3333)
  line L336 (0.8333, -6.25) -> (0.8333, -6.4583)
  line L337 (0.8333, -6.4583) -> (0.625, -6.4583)
  line L338 (0.625, -6.4583) -> (0.625, -6.6667)
  line L339 (0.625, -6.6667) -> (0.4167, -6.6667)
  line L340 (0.4167, -6.6667) -> (0.4167, -6.875)
  line L341 (0.4167, -6.875) -> (0.2083, -6.875)
  line L342 (0.2083, -6.875) -> (0.2083, -7.0833)
  line L343 (0.2083, -7.0833) -> (0, -7.0833)
  line L344 (0, -7.0833) -> (0, -9.1667)
  line L345 (0, -9.1667) -> (0.2083, -9.1667)
  line L346 (0.2083, -9.1667) -> (0.2083, -9.375)
  line L347 (0.2083, -9.375) -> (0.4167, -9.375)
  line L348 (0.4167, -9.375) -> (0.4167, -9.5833)
  line L349 (0.4167, -9.5833) -> (0.625, -9.5833)
  line L350 (0.625, -9.5833) -> (0.625, -9.7917)
  line L351 (0.625, -9.7917) -> (0.8333, -9.7917)
  line L352 (0.8333, -9.7917) -> (0.8333, -10)
  line L353 (0.8333, -10) -> (2.2917, -10)
  line L354 (2.2917, -10) -> (2.2917, -9.7917)
  line L355 (2.2917, -9.7917) -> (2.5, -9.7917)
  line L356 (2.5, -9.7917) -> (2.5, -9.5833)
  line L357 (2.5, -9.5833) -> (2.7083, -9.5833)
  line L358 (2.7083, -9.5833) -> (2.7083, -9.375)
  line L359 (2.7083, -9.375) -> (2.9167, -9.375)
  line L360 (2.9167, -9.375) -> (2.9167, -7.7083)
  line L361 (2.9167, -7.7083) -> (1.4583, -7.7083)
  line L362 (1.4583, -7.7083) -> (1.4583, -8.5417)
  line L363 (1.4583, -8.5417) -> (2.2917, -8.5417)
  line L364 (2.2917, -8.5417) -> (2.2917, -8.75)
  line L365 (2.2917, -8.75) -> (2.0833, -8.75)
  line L366 (2.0833, -8.75) -> (2.0833, -8.9583)
  line L367 (2.0833, -8.9583) -> (1.875, -8.9583)
  line L368 (1.875, -8.9583) -> (1.875, -9.1667)
  line L369 (1.875, -9.1667) -> (1.25, -9.1667)
  line L370 (1.25, -9.1667) -> (1.25, -8.9583)
  line L371 (1.25, -8.9583) -> (1.0417, -8.9583)
  line L372 (1.0417, -8.9583) -> (1.0417, -8.75)
  line L373 (1.0417, -8.75) -> (0.8333, -8.75)
  line L374 (0.8333, -8.75) -> (0.8333, -7.5)
  line L375 (0.8333, -7.5) -> (1.0417, -7.5)
  line L376 (1.0417, -7.5) -> (1.0417, -7.2917)
  line L377 (1.0417, -7.2917) -> (1.25, -7.2917)
  line L378 (1.25, -7.2917) -> (1.25, -7.0833)
  line L379 (1.25, -7.0833) -> (2.2917, -7.0833)
  line L380 (2.2917, -7.0833) -> (2.2917, -6.25)
  line L381 (2.2917, -6.25) -> (0.8333, -6.25)
  line L382 (4.5833, -6.25) -> (4.5833, -6.4583)
  line L383 (4.5833, -6.4583) -> (4.375, -6.4583)
  line L384 (4.375, -6.4583) -> (4.375, -6.6667)
  line L385 (4.375, -6.6667) -> (4.1667, -6.6667)
  line L386 (4.1667, -6.6667) -> (4.1667, -6.875)
  line L387 (4.1667, -6.875) -> (3.9583, -6.875)
  line L388 (3.9583, -6.875) -> (3.9583, -7.0833)
  line L389 (3.9583, -7.0833) -> (3.75, -7.0833)
  line L390 (3.75, -7.0833) -> (3.75, -10)
  line L391 (3.75, -10) -> (4.5833, -10)
  line L392 (4.5833, -10) -> (4.5833, -9.1667)
  line L393 (4.5833, -9.1667) -> (5.2083, -9.1667)
  line L394 (5.2083, -9.1667) -> (5.2083, -10)
  line L395 (5.2083, -10) -> (6.0417, -10)
  line L396 (6.0417, -10) -> (6.0417, -7.0833)
  line L397 (6.0417, -7.0833) -> (5.8333, -7.0833)
  line L398 (5.8333, -7.0833) -> (5.8333, -6.875)
  line L399 (5.8333, -6.875) -> (5.625, -6.875)
  line L400 (5.625, -6.875) -> (5.625, -6.6667)
  line L401 (5.625, -6.6667) -> (5.4167, -6.6667)
  line L402 (5.4167, -6.6667) -> (5.4167, -6.4583)
  line L403 (5.4167, -6.4583) -> (5.2083, -6.4583)
  line L404 (5.2083, -6.4583) -> (5.2083, -6.25)
  line L405 (5.2083, -6.25) -> (4.5833, -6.25)
  line L406 (7.5, -6.25) -> (7.5, -6.4583)
  line L407 (7.5, -6.4583) -> (7.2917, -6.4583)
  line L408 (7.2917, -6.4583) -> (7.2917, -6.6667)
  line L409 (7.2917, -6.6667) -> (7.0833, -6.6667)
  line L410 (7.0833, -6.6667) -> (7.0833, -6.875)
  line L411 (7.0833, -6.875) -> (6.875, -6.875)
  line L412 (6.875, -6.875) -> (6.875, -7.0833)
  line L413 (6.875, -7.0833) -> (6.6667, -7.0833)
  line L414 (6.6667, -7.0833) -> (6.6667, -10)
  line L415 (6.6667, -10) -> (7.5, -10)
  line L416 (7.5, -10) -> (7.5, -7.5)
  line L417 (7.5, -7.5) -> (7.7083, -7.5)
  line L418 (7.7083, -7.5) -> (7.7083, -7.2917)
  line L419 (7.7083, -7.2917) -> (8.125, -7.2917)
  line L420 (8.125, -7.2917) -> (8.125, -7.5)
  line L421 (8.125, -7.5) -> (8.3333, -7.5)
  line L422 (8.3333, -7.5) -> (8.3333, -8.5417)
  line L423 (8.3333, -8.5417) -> (8.9583, -8.5417)
  line L424 (8.9583, -8.5417) -> (8.9583, -7.5)
  line L425 (8.9583, -7.5) -> (9.1667, -7.5)
  line L426 (9.1667, -7.5) -> (9.1667, -7.2917)
  line L427 (9.1667, -7.2917) -> (9.5833, -7.2917)
  line L428 (9.5833, -7.2917) -> (9.5833, -7.5)
  line L429 (9.5833, -7.5) -> (9.7917, -7.5)
  line L430 (9.7917, -7.5) -> (9.7917, -10)
  line L431 (9.7917, -10) -> (10.625, -10)
  line L432 (10.625, -10) -> (10.625, -7.0833)
  line L433 (10.625, -7.0833) -> (10.4167, -7.0833)
  line L434 (10.4167, -7.0833) -> (10.4167, -6.875)
  line L435 (10.4167, -6.875) -> (10.2083, -6.875)
  line L436 (10.2083, -6.875) -> (10.2083, -6.6667)
  line L437 (10.2083, -6.6667) -> (10, -6.6667)
  line L438 (10, -6.6667) -> (10, -6.4583)
  line L439 (10, -6.4583) -> (9.7917, -6.4583)
  line L440 (9.7917, -6.4583) -> (9.7917, -6.25)
  line L441 (9.7917, -6.25) -> (8.9583, -6.25)
  line L442 (8.9583, -6.25) -> (8.9583, -6.4583)
  line L443 (8.9583, -6.4583) -> (8.75, -6.4583)
  line L444 (8.75, -6.4583) -> (8.75, -6.6667)
  line L445 (8.75, -6.6667) -> (8.5417, -6.6667)
  line L446 (8.5417, -6.6667) -> (8.5417, -6.4583)
  line L447 (8.5417, -6.4583) -> (8.3333, -6.4583)
  line L448 (8.3333, -6.4583) -> (8.3333, -6.25)
  line L449 (8.3333, -6.25) -> (7.5, -6.25)
  line L450 (11.25, -6.25) -> (11.25, -10)
  line L451 (11.25, -10) -> (13.5417, -10)
  line L452 (13.5417, -10) -> (13.5417, -9.1667)
  line L453 (13.5417, -9.1667) -> (12.0833, -9.1667)
  line L454 (12.0833, -9.1667) -> (12.0833, -8.5417)
  line L455 (12.0833, -8.5417) -> (12.7083, -8.5417)
  line L456 (12.7083, -8.5417) -> (12.7083, -7.7083)
  line L457 (12.7083, -7.7083) -> (12.0833, -7.7083)
  line L458 (12.0833, -7.7083) -> (12.0833, -7.0833)
  line L459 (12.0833, -7.0833) -> (13.5417, -7.0833)
  line L460 (13.5417, -7.0833) -> (13.5417, -6.25)
  line L461 (13.5417, -6.25) -> (11.25, -6.25)
  line L462 (15, -6.25) -> (15, -6.4583)
  line L463 (15, -6.4583) -> (14.7917, -6.4583)
  line L464 (14.7917, -6.4583) -> (14.7917, -6.6667)
  line L465 (14.7917, -6.6667) -> (14.5833, -6.6667)
  line L466 (14.5833, -6.6667) -> (14.5833, -6.875)
  line L467 (14.5833, -6.875) -> (14.375, -6.875)
  line L468 (14.375, -6.875) -> (14.375, -7.7083)
  line L469 (14.375, -7.7083) -> (14.5833, -7.7083)
  line L470 (14.5833, -7.7083) -> (14.5833, -7.9167)
  line L471 (14.5833, -7.9167) -> (14.7917, -7.9167)
  line L472 (14.7917, -7.9167) -> (14.7917, -8.125)
  line L473 (14.7917, -8.125) -> (15, -8.125)
  line L474 (15, -8.125) -> (15, -8.3333)
  line L475 (15, -8.3333) -> (15.2083, -8.3333)
  line L476 (15.2083, -8.3333) -> (15.2083, -8.5417)
  line L477 (15.2083, -8.5417) -> (16.0417, -8.5417)
  line L478 (16.0417, -8.5417) -> (16.0417, -8.75)
  line L479 (16.0417, -8.75) -> (16.25, -8.75)
  line L480 (16.25, -8.75) -> (16.25, -9.1667)
  line L481 (16.25, -9.1667) -> (14.375, -9.1667)
  line L482 (14.375, -9.1667) -> (14.375, -10)
  line L483 (14.375, -10) -> (16.6667, -10)
  line L484 (16.6667, -10) -> (16.6667, -9.7917)
  line L485 (16.6667, -9.7917) -> (16.875, -9.7917)
  line L486 (16.875, -9.7917) -> (16.875, -9.5833)
  line L487 (16.875, -9.5833) -> (17.0833, -9.5833)
  line L488 (17.0833, -9.5833) -> (17.0833, -9.375)
  line L489 (17.0833, -9.375) -> (17.2917, -9.375)
  line L490 (17.2917, -9.375) -> (17.2917, -8.5417)
  line L491 (17.2917, -8.5417) -> (17.0833, -8.5417)
  line L492 (17.0833, -8.5417) -> (17.0833, -8.3333)
  line L493 (17.0833, -8.3333) -> (16.875, -8.3333)
  line L494 (16.875, -8.3333) -> (16.875, -8.125)
  line L495 (16.875, -8.125) -> (16.6667, -8.125)
  line L496 (16.6667, -8.125) -> (16.6667, -7.9167)
  line L497 (16.6667, -7.9167) -> (16.4583, -7.9167)
  line L498 (16.4583, -7.9167) -> (16.4583, -7.7083)
  line L499 (16.4583, -7.7083) -> (15.625, -7.7083)
  line L500 (15.625, -7.7083) -> (15.625, -7.5)
  line L501 (15.625, -7.5) -> (15.4167, -7.5)
  line L502 (15.4167, -7.5) -> (15.4167, -7.0833)
  line L503 (15.4167, -7.0833) -> (17.2917, -7.0833)
  line L504 (17.2917, -7.0833) -> (17.2917, -6.25)
  line L505 (17.2917, -6.25) -> (15, -6.25)
  line L506 (2.0833, -6.4583) -> (2.0833, -6.875)
  line L507 (2.0833, -6.875) -> (1.0417, -6.875)
  line L508 (1.0417, -6.875) -> (1.0417, -7.0833)
  line L509 (1.0417, -7.0833) -> (0.8333, -7.0833)
  line L510 (0.8333, -7.0833) -> (0.8333, -7.2917)
  line L511 (0.8333, -7.2917) -> (0.625, -7.2917)
  line L512 (0.625, -7.2917) -> (0.625, -8.9583)
  line L513 (0.625, -8.9583) -> (0.8333, -8.9583)
  line L514 (0.8333, -8.9583) -> (0.8333, -9.1667)
  line L515 (0.8333, -9.1667) -> (1.0417, -9.1667)
  line L516 (1.0417, -9.1667) -> (1.0417, -9.375)
  line L517 (1.0417, -9.375) -> (2.0833, -9.375)
  line L518 (2.0833, -9.375) -> (2.0833, -9.1667)
  line L519 (2.0833, -9.1667) -> (2.2917, -9.1667)
  line L520 (2.2917, -9.1667) -> (2.2917, -8.9583)
  line L521 (2.2917, -8.9583) -> (2.5, -8.9583)
  line L522 (2.5, -8.9583) -> (2.5, -8.3333)
  line L523 (2.5, -8.3333) -> (1.6667, -8.3333)
  line L524 (1.6667, -8.3333) -> (1.6667, -7.9167)
  line L525 (1.6667, -7.9167) -> (2.7083, -7.9167)
  line L526 (2.7083, -7.9167) -> (2.7083, -9.1667)
  line L527 (2.7083, -9.1667) -> (2.5, -9.1667)
  line L528 (2.5, -9.1667) -> (2.5, -9.375)
  line L529 (2.5, -9.375) -> (2.2917, -9.375)
  line L530 (2.2917, -9.375) -> (2.2917, -9.5833)
  line L531 (2.2917, -9.5833) -> (2.0833, -9.5833)
  line L532 (2.0833, -9.5833) -> (2.0833, -9.7917)
  line L533 (2.0833, -9.7917) -> (1.0417, -9.7917)
  line L534 (1.0417, -9.7917) -> (1.0417, -9.5833)
  line L535 (1.0417, -9.5833) -> (0.8333, -9.5833)
  line L536 (0.8333, -9.5833) -> (0.8333, -9.375)
  line L537 (0.8333, -9.375) -> (0.625, -9.375)
  line L538 (0.625, -9.375) -> (0.625, -9.1667)
  line L539 (0.625, -9.1667) -> (0.4167, -9.1667)
  line L540 (0.4167, -9.1667) -> (0.4167, -8.9583)
  line L541 (0.4167, -8.9583) -> (0.2083, -8.9583)
  line L542 (0.2083, -8.9583) -> (0.2083, -7.2917)
  line L543 (0.2083, -7.2917) -> (0.4167, -7.2917)
  line L544 (0.4167, -7.2917) -> (0.4167, -7.0833)
  line L545 (0.4167, -7.0833) -> (0.625, -7.0833)
  line L546 (0.625, -7.0833) -> (0.625, -6.875)
  line L547 (0.625, -6.875) -> (0.8333, -6.875)
  line L548 (0.8333, -6.875) -> (0.8333, -6.6667)
  line L549 (0.8333, -6.6667) -> (1.0417, -6.6667)
  line L550 (1.0417, -6.6667) -> (1.0417, -6.4583)
  line L551 (1.0417, -6.4583) -> (2.0833, -6.4583)
  line L552 (5, -6.4583) -> (5, -6.6667)
  line L553 (5, -6.6667) -> (5.2083, -6.6667)
  line L554 (5.2083, -6.6667) -> (5.2083, -6.875)
  line L555 (5.2083, -6.875) -> (5.4167, -6.875)
  line L556 (5.4167, -6.875) -> (5.4167, -7.0833)
  line L557 (5.4167, -7.0833) -> (5.625, -7.0833)
  line L558 (5.625, -7.0833) -> (5.625, -7.2917)
  line L559 (5.625, -7.2917) -> (5.8333, -7.2917)
  line L560 (5.8333, -7.2917) -> (5.8333, -9.7917)
  line L561 (5.8333, -9.7917) -> (5.4167, -9.7917)
  line L562 (5.4167, -9.7917) -> (5.4167, -8.9583)
  line L563 (5.4167, -8.9583) -> (4.375, -8.9583)
  line L564 (4.375, -8.9583) -> (4.375, -9.7917)
  line L565 (4.375, -9.7917) -> (3.9583, -9.7917)
  line L566 (3.9583, -9.7917) -> (3.9583, -7.2917)
  line L567 (3.9583, -7.2917) -> (4.1667, -7.2917)
  line L568 (4.1667, -7.2917) -> (4.1667, -7.0833)
  line L569 (4.1667, -7.0833) -> (4.375, -7.0833)
  line L570 (4.375, -7.0833) -> (4.375, -6.875)
  line L571 (4.375, -6.875) -> (4.5833, -6.875)
  line L572 (4.5833, -6.875) -> (4.5833, -6.6667)
  line L573 (4.5833, -6.6667) -> (4.7917, -6.6667)
  line L574 (4.7917, -6.6667) -> (4.7917, -6.4583)
  line L575 (4.7917, -6.4583) -> (5, -6.4583)
  line L576 (8.125, -6.4583) -> (8.125, -6.6667)
  line L577 (8.125, -6.6667) -> (8.3333, -6.6667)
  line L578 (8.3333, -6.6667) -> (8.3333, -6.875)
  line L579 (8.3333, -6.875) -> (8.5417, -6.875)
  line L580 (8.5417, -6.875) -> (8.5417, -7.0833)
  line L581 (8.5417, -7.0833) -> (8.75, -7.0833)
  line L582 (8.75, -7.0833) -> (8.75, -6.875)
  line L583 (8.75, -6.875) -> (8.9583, -6.875)
  line L584 (8.9583, -6.875) -> (8.9583, -6.6667)
  line L585 (8.9583, -6.6667) -> (9.1667, -6.6667)
  line L586 (9.1667, -6.6667) -> (9.1667, -6.4583)
  line L587 (9.1667, -6.4583) -> (9.5833, -6.4583)
  line L588 (9.5833, -6.4583) -> (9.5833, -6.6667)
  line L589 (9.5833, -6.6667) -> (9.7917, -6.6667)
  line L590 (9.7917, -6.6667) -> (9.7917, -6.875)
  line L591 (9.7917, -6.875) -> (10, -6.875)
  line L592 (10, -6.875) -> (10, -7.0833)
  line L593 (10, -7.0833) -> (10.2083, -7.0833)
  line L594 (10.2083, -7.0833) -> (10.2083, -7.2917)
  line L595 (10.2083, -7.2917) -> (10.4167, -7.2917)
  line L596 (10.4167, -7.2917) -> (10.4167, -9.7917)
  line L597 (10.4167, -9.7917) -> (10, -9.7917)
  line L598 (10, -9.7917) -> (10, -7.2917)
  line L599 (10, -7.2917) -> (9.7917, -7.2917)
  line L600 (9.7917, -7.2917) -> (9.7917, -7.0833)
  line L601 (9.7917, -7.0833) -> (9.5833, -7.0833)
  line L602 (9.5833, -7.0833) -> (9.5833, -6.875)
  line L603 (9.5833, -6.875) -> (9.1667, -6.875)
  line L604 (9.1667, -6.875) -> (9.1667, -7.0833)
  line L605 (9.1667, -7.0833) -> (8.9583, -7.0833)
  line L606 (8.9583, -7.0833) -> (8.9583, -7.2917)
  line L607 (8.9583, -7.2917) -> (8.75, -7.2917)
  line L608 (8.75, -7.2917) -> (8.75, -8.3333)
  line L609 (8.75, -8.3333) -> (8.5417, -8.3333)
  line L610 (8.5417, -8.3333) -> (8.5417, -7.2917)
  line L611 (8.5417, -7.2917) -> (8.3333, -7.2917)
  line L612 (8.3333, -7.2917) -> (8.3333, -7.0833)
  line L613 (8.3333, -7.0833) -> (8.125, -7.0833)